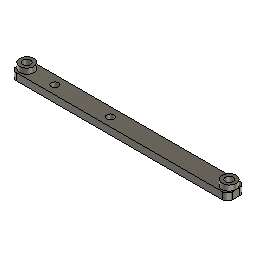
duet2deux-side-mount (Autodesk Fusion 360 design; units mm, degrees)
Autodesk Fusion 360 part; units mm, degrees
sketch "Sketch1" plane through (0, 0, 0) normal (0, 0, 1) x (1, 0, 0)
  circle A0 centre (-41.5, 0) radius 1.2
  circle A1 centre (-10, 0) radius 1.2
  circle A2 centre (-10, 0) radius 2
  circle A3 centre (-57.5, 0) radius 2.2
  circle A4 centre (57.5, 0) radius 2.2
  line L0 (-57.5, 0) -> (57.5, 0) construction
  circle A5 centre (-41.5, 0) radius 2
  line L1 (-58.5, 5) -> (58.5, 5)
  line L2 (61.5, 2) -> (61.5, -2)
  line L3 (58.5, -5) -> (-58.5, -5)
  line L4 (-61.5, -2) -> (-61.5, 2)
  line L5 (0, 5) -> (0, -5) construction
  arc A6 (-58.5, 5) -> (-61.5, 2) centre (-58.5, 2) ccw
  arc A7 (-61.5, -2) -> (-58.5, -5) centre (-58.5, -2) ccw
  arc A8 (58.5, -5) -> (61.5, -2) centre (58.5, -2) ccw
  arc A9 (61.5, 2) -> (58.5, 5) centre (58.5, 2) ccw
  circle A10 centre (-57.5, 0) radius 4
  circle A11 centre (57.5, 0) radius 4
  point P0 (-8.9196, -41.0353)
  point P1 (61.5, -5)
  point P2 (-61.5, -5)
  dimension "d1" = 2.4
  dimension "d3" = 2.4
  dimension "d4" = 4
  dimension "d6" = 4.4
  dimension "d7" = 4.4
  dimension "d11" = 115
  dimension "d14" = 4
  dimension "d15" = 31.5
  dimension "d16" = 123
  dimension "d17" = 10
  dimension "d18" = 3
  dimension "d23" = 8
  dimension "d24" = 8
  dimension "d27" = 20
  constraint concentric A1 A2
  constraint coincident A3.centre L0.start
  constraint horizontal L0
  constraint coincident A4.centre L0.end
  constraint concentric A0 A5
  constraint coincident L0 A0.centre
  constraint coincident A1.centre L0
  constraint horizontal L1
  constraint vertical L2
  constraint horizontal L3
  constraint vertical L4
  constraint midpoint L0 origin
  constraint coincident L5 origin
  constraint midpoint L5 origin
  constraint coincident L1 L5.start
  constraint tangent L1 A6
  constraint tangent L4 A6
  constraint coincident L3 L5.end
  constraint coincident P2 L3
  constraint coincident P2 L4
  constraint tangent L3 A7
  constraint tangent L4 A7
  constraint equal A6 A7
  constraint coincident P1 L2
  constraint coincident P1 L3
  constraint tangent L2 A8
  constraint tangent L3 A8
  constraint equal A6 A8
  constraint tangent L1 A9
  constraint tangent L2 A9
  constraint equal A6 A9
  constraint concentric A3 A10
  constraint concentric A4 A11
  constraint tangent L4 A10
  measures "d1" diameter of A0
  measures "d3" diameter of A1
  measures "d4" diameter of A2
  measures "d6" diameter of A3
  measures "d7" diameter of A4
  measures "d11" distance of A3.centre A4.centre
  measures "d14" diameter of A5
  measures "d15" horizontal distance of A1.centre A0.centre
  measures "d16" distance of P1 P2
  measures "d17" distance of L1 L3
  measures "d18" radius of A6
  measures "d23" diameter of A10
  measures "d24" diameter of A11
  measures "d27" distance of A0.centre L4
extrude "Extrude1" add sketch "Sketch1" along normal blind 4 contours A10 | A11 | L1 L2 L3 L4 A6 A7 A8 A9
extrude "Extrude2" add sketch "Sketch1" along normal blind 1 contours A2 | A5
extrude "Extrude3" add sketch "Sketch1" along normal blind 7 contours A10 | A11
